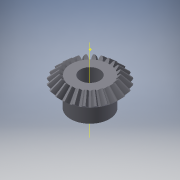
# Autodesk Inventor part: Bevel Gear2
Saved by Autodesk Inventor 2016 (Build 200138000, 138)
## iProperties
Created: 2015-06-13
Part Number: Bevel Gear2
Material: Steel, Mild
Document SubType Name: Modeling
Designer: steele
Categories: <?xml version="1.0" encoding="UTF-16"?> <MemberInstance><Categories><FamilyTemplate><FamilyTemplateParameter ValueType="xs:double" Id="1" ObjectReferenceKey="da_z" ObjectType="kUserParameterObject"/><FamilyTemplateParameter ValueType="xs:double" Id="2" ObjectReferenceKey="da_b" ObjectType="kUserParameterObject"/><FamilyTemplateParameter ValueType="xs:double" Id="3" ObjectReferenceKey="da_beta" ObjectType="kUserParameterObject"/><FamilyTemplateParameter ValueType="xs:double" Id="4" ObjectReferenceKey="da_dae" ObjectType="kUserParameterObject"/><FamilyTemplateParameter ValueType="xs:double" Id="5" ObjectReferenceKey="da_ve" ObjectType="kUserParameterObject"/><FamilyTemplateParameter ValueType="xs:double" Id="6" ObjectReferenceKey="da_omega" ObjectType="kUserParameterObject"/><FamilyTemplateParameter ValueType="xs:string" Id="7" ObjectReferenceKey="EAIAABAAAAAAHwAAAAAAAIAAAAAAAAAA" ObjectType="83914240" SubObjectId="SurfaceGeometry"/></FamilyTemplate><ParamToTemplateMap><ParamToTemplate CategoryParameter="//CategoryParameter[@InternalName='046C89C9-8512-4d59-83FE-43B91F4F132A']" TemplateParameter="1"/><ParamToTemplate CategoryParameter="//CategoryParameter[@InternalName='2552DF32-E462-4b46-AEBF-C6C7768E72AC']" TemplateParameter="2"/><ParamToTemplate CategoryParameter="//CategoryParameter[@InternalName='C9EE641D-15FC-4fae-A226-E94C4372FDD7']" TemplateParameter="3"/><ParamToTemplate><ParamToTemplate CategoryParameter="//CategoryParameter[@InternalName='00B6519A-459B-49c7-AD84-2E56D39A5744']" ConstantValue="-0.000000"/></ParamToTemplate><ParamToTemplate><ParamToTemplate CategoryParameter="//CategoryParameter[@InternalName='04B31F0E-C7A6-4894-AA32-9629BEFACF47']" ConstantValue="1.000000"/></ParamToTemplate><ParamToTemplate><ParamToTemplate CategoryParameter="//CategoryParameter[@InternalName='43CBEC2E-7847-49e7-A936-2F7889FCB2D9']" ConstantValue="0.200000"/></ParamToTemplate><ParamToTemplate><ParamToTemplate CategoryParameter="//CategoryParameter[@InternalName='B1EFC894-105D-4ebd-86BF-FA20ED196853']" ConstantValue="0.300000"/></ParamToTemplate><ParamToTemplate><ParamToTemplate CategoryParameter="//CategoryParameter[@InternalName='51175063-3D10-4879-93E8-6246FE8B403D']" ConstantValue="2061532430.657340"/></ParamToTemplate><ParamToTemplate><ParamToTemplate CategoryParameter="//CategoryParameter[@InternalName='A3A52E27-4454-46a9-B0BD-C932399B70AF']" ConstantValue="0.300000"/></ParamToTemplate><ParamToTemplate CategoryParameter="//CategoryParameter[@InternalName='2A200944-5A8C-41ca-B96E-8520D2E510F1']" TemplateParameter="4"/><ParamToTemplate><ParamToTemplate CategoryParameter="//CategoryParameter[@InternalName='1A637F62-92C8-44bc-B81F-10802510B579']" ConstantValue="2.855338"/></ParamToTemplate><ParamToTemplate CategoryParameter="//CategoryParameter[@InternalName='B52DD4BE-6863-48fb-BF58-89EF6F9EC65C']" TemplateParameter="5"/><ParamToTemplate><ParamToTemplate CategoryParameter="//CategoryParameter[@InternalName='3956BFF2-84D2-457d-93C2-9B0613DEBA67']" ConstantValue="1.268779"/></ParamToTemplate><ParamToTemplate CategoryParameter="//CategoryParameter[@InternalName='739CFA02-461B-4bf8-8049-181FCAD8B28F']" TemplateParameter="6"/><ParamToTemplate><ParamToTemplate CategoryParameter="//CategoryParameter[@InternalName='A27E999F-E2CE-4481-8A2A-EBF499C4C3C5']" ConstantValue="-0.000000"/></ParamToTemplate><ParamToTemplate><ParamToTemplate CategoryParameter="//CategoryParameter[@InternalName='9E1B4470-B2D3-4ff1-B813-535BB4CDF51A']" ConstantValue="3523220.976809"/></ParamToTemplate><ParamToTemplate><ParamToTemplate CategoryParameter="//CategoryParameter[@InternalName='F8452263-BFF6-458c-9FB1-07C4B99E95CD']" ConstantValue="11397033.805607"/></ParamToTemplate><ParamToTemplate><ParamToTemplate CategoryParameter="//CategoryParameter[@InternalName='3E3BB259-FD49-497f-8171-6EBC954A3479']" ConstantValue="2.000000"/></ParamToTemplate><ParamToTemplate CategoryParameter="//CategoryParameter[@InternalName='27C3BAF2-7550-4e4b-AE2C-0DB134B7D9B7']" TemplateParameter="7"/></ParamToTemplateMap><Category DisplayName="Gear" InternalName="DC85795E-93AB-48d5-8EEE-5A27447B64BD" Mnemonic="Gear"><CategoryParameter DisplayName="z" InternalName="046C89C9-8512-4d59-83FE-43B91F4F132A" Mnemonic="z"/><CategoryParameter DisplayName="b" InternalName="2552DF32-E462-4b46-AEBF-C6C7768E72AC" Mnemonic="b"/><CategoryParameter DisplayName="||b|" InternalName="C9EE641D-15FC-4fae-A226-E94C4372FDD7" Mnemonic="beta"/><CategoryParameter DisplayName="x" InternalName="00B6519A-459B-49c7-AD84-2E56D39A5744" Mnemonic="x"/><CategoryParameter DisplayName="a*" InternalName="04B31F0E-C7A6-4894-AA32-9629BEFACF47" Mnemonic="a"/><CategoryParameter DisplayName="c*" InternalName="43CBEC2E-7847-49e7-A936-2F7889FCB2D9" Mnemonic="c"/><CategoryParameter DisplayName="r|.f|*" InternalName="B1EFC894-105D-4ebd-86BF-FA20ED196853" Mnemonic="rf"/><CategoryParameter DisplayName="E" InternalName="51175063-3D10-4879-93E8-6246FE8B403D" Mnemonic="E"/><CategoryParameter DisplayName="||m|" InternalName="A3A52E27-4454-46a9-B0BD-C932399B70AF" Mnemonic="mi"/><Category DisplayName="BevelGear" InternalName="0C98F69A-0C2B-4791-B2FE-7691BB227E77" Mnemonic="BevelGear"><CategoryParameter DisplayName="d|.ae|" InternalName="2A200944-5A8C-41ca-B96E-8520D2E510F1" Mnemonic="dae"/><CategoryParameter DisplayName="d|.ai|" InternalName="1A637F62-92C8-44bc-B81F-10802510B579" Mnemonic="dai"/><CategoryParameter DisplayName="A|.e|" InternalName="B52DD4BE-6863-48fb-BF58-89EF6F9EC65C" Mnemonic="ve"/><CategoryParameter DisplayName="A|.i|" InternalName="3956BFF2-84D2-457d-93C2-9B0613DEBA67" Mnemonic="vi"/><CategoryParameter DisplayName="||S|" InternalName="739CFA02-461B-4bf8-8049-181FCAD8B28F" Mnemonic="omega"/><CategoryParameter DisplayName="x|.t|" InternalName="A27E999F-E2CE-4481-8A2A-EBF499C4C3C5" Mnemonic="xt"/><CategoryParameter DisplayName="||s||.Flim|" InternalName="9E1B4470-B2D3-4ff1-B813-535BB4CDF51A" Mnemonic="sFlim"/><CategoryParameter DisplayName="||s||.Hlim|" InternalName="F8452263-BFF6-458c-9FB1-07C4B99E95CD" Mnemonic="sHlim"/><CategoryParameter DisplayName="type" InternalName="3E3BB259-FD49-497f-8171-6EBC954A3479" Mnemonic="type"/><CategoryParameter DisplayName="PitchDiameter" InternalName="27C3BAF2-7550-4e4b-AE2C-0DB134B7D9B7" Mnemonic="IDS_PITCHDIAM"/></Category></Category></Categories></MemberInstance>
Mass: 60.9118 g
Surface Area: 34.3074 cm^2
Volume: 7.7496 cm^3
Density: 7.86 g/cm^3
Appearance: Steel
CustomPartVersion: 1
d48: 0.0000 in
d49: 0.0000 in
d50: 90.00 deg
d52: 0.0000 in
d53: 0.0000 in
d54: 0.00 deg
Author: steele
Autodesk Inventor part; units mm, degrees
ref_plane "Mesh Plane2" through (0, 0, 0) normal (0.9914449, 0.1305262, 0) x (0, 0, 1)
sketch "Teeth Body Sketch" plane through (0, 0, 0) normal (1, 0, 0) x (0, 1, 0)
  line L0 (0, 0) -> (17.702962, -20.397039) construction
  line L1 (17.702962, -20.397039) -> (20.172532, -17.927468)
  line L2 (20.172532, -17.927468) -> (0, 0) construction
  line L3 (19.05, -19.05) -> (0, 0) construction
  line L4 (12.528903, -14.43558) -> (14.27669, -12.687793)
  line L5 (17.702962, -20.397039) -> (12.528903, -14.43558)
  line L6 (20.172532, -17.927468) -> (14.27669, -12.687793)
  line L7 (0, -33.066314) -> (0, 5.511052)
  line L8 (0, -19.05) -> (20.172532, -19.05) construction
  dimension "d0" = 38.1
  dimension "d1" = 35.40592
  dimension "d2" = 40.34506
  dimension "d3" = 7.874
  dimension "d4" = 17.92747
  constraints: 16 end point, 4 point on line, 3 perpendicular, 2 collinear, 1 horizontal alignment, 1 vertical alignment
  measures "d0" diameter of L3.start L7
  measures "d1" diameter of L0.end L7
  measures "d2" diameter of L1.end L7
  measures "d3" distance between parallel lines of L1 L4
  measures "d4" vertical distance of L1.end L0.start
revolve "Teeth Body" add sketch "Teeth Body Sketch" angle 360 about axis through (0, 0, 0) along (0, 0, 1)
ref_plane "Tooth Plane" through (0, 19.05, -19.05) normal (0, -0.7071068, 0.7071068) x (1, 0, 0)
sketch "Start Sketch" plane through (0, 19.05, -19.05) normal (0, -0.7071068, 0.7071068) x (1, 0, 0)
  line L0 (0, -43.954783) -> (0, 12.281529)
  arc A0 (-0.600729, -2.3241) -> (-2.796445, 2.50275) centre (-10.245884, -3.798809) ccw
  arc A1 (2.796445, 2.50275) -> (0.600729, -2.3241) centre (10.245884, -3.798809) ccw
  line L1 (-0.600729, -2.3241) -> (0.600729, -2.3241)
  arc A2 (2.796445, 2.50275) -> (-2.796445, 2.50275) centre (0, -26.940768) ccw
  dimension "d7" = 9.75724
  dimension "d8" = 10.24588
  dimension "d9" = 23.14196
  dimension "d57" = 29.57602
  dimension "d58" = 24.61667
  constraints: 6 point on circle, 3 centre point, 3 symmetric about line, 2 end point, 1 coincident, 1 perpendicular, 1 other
  measures "d7" radius of A0
  measures "d8" horizontal distance of point (0, -26.941) A0.centre
  measures "d9" vertical distance of point (0, -26.941) A0.centre
  measures "d57" radius of A2
  measures "d58" distance from line of A2.centre L1
sketch "End Sketch" plane through (0, 13.358763, -13.358763) normal (0, -0.7071068, 0.7071068) x (1, 0, 0)
  line L0 (0, -28.080566) -> (0, 7.892027)
  arc A0 (-0.42186, -1.605152) -> (-1.963796, 1.78449) centre (-7.195145, -2.640763) ccw
  arc A1 (1.963796, 1.78449) -> (0.42186, -1.605152) centre (7.195145, -2.640763) ccw
  line L1 (-0.42186, -1.605152) -> (0.42186, -1.605152)
  arc A2 (1.963796, 1.78449) -> (-1.963796, 1.78449) centre (0, -18.892143) ccw
  dimension "d12" = 6.852
  dimension "d15" = 7.19514
  dimension "d16" = 16.25138
  dimension "d59" = 20.76968
  dimension "d60" = 17.28699
  constraints: 6 point on circle, 3 centre point, 3 symmetric about line, 2 end point, 1 coincident, 1 other
  measures "d12" radius of A0
  measures "d15" horizontal distance of A0.centre point (0, -18.892)
  measures "d16" vertical distance of A0.centre point (0, -18.892)
  measures "d59" radius of A2
  measures "d60" distance from line of A2.centre L1
loft "Loft" cut profiles "Start Sketch", "End Sketch"
pattern_circular "Circular Pattern" count 24 over 360 about axis through (0, 0, 0) along (0, 0, 1) of "Loft"
ref_plane "End Plane" through (0, 13.358763, -13.358763) normal (0, -0.7071068, 0.7071068) x (1, 0, 0)
sketch3d "3D Sketch Right"
ref_plane "End Plane Right" through (-1.865438, 13.227875, -13.358763) normal (0.0987415, -0.7001786, 0.7071068) x (0.9902021, 0.1396415, 0)
sketch "End Sketch Right" plane through (-1.865438, 13.227875, -13.358763) normal (0.0987415, -0.7001786, 0.7071068) x (0.9902021, 0.1396415, 0)
  arc A0 (-0.42186, -1.605152) -> (-1.963796, 1.78449) centre (-7.195145, -2.640763) ccw
  line L0 (0, -30.54214) -> (0, 10.353601)
  arc A1 (1.963796, 1.78449) -> (0.42186, -1.605152) centre (7.195145, -2.640763) ccw
  line L1 (-0.42186, -1.605152) -> (0.42186, -1.605152)
  arc A2 (1.963796, 1.78449) -> (-1.963796, 1.78449) centre (0, -18.892143) ccw
  dimension "d70" = 7.19514
  dimension "d71" = 16.25138
  dimension "d72" = 6.852
  dimension "d73" = 17.28699
  dimension "d74" = 20.76968
  constraints: 6 point on circle, 3 centre point, 3 symmetric about line, 2 end point, 1 coincident, 1 perpendicular, 1 other
  measures "d70" horizontal distance of A2.centre A0.centre
  measures "d71" vertical distance of point (0, -18.892) A0.centre
  measures "d72" radius of A0
  measures "d73" distance from line of point (0, -18.892) L1
  measures "d74" radius of A2
feature "Loft Right" [suppressed]
pattern_circular "Circular Pattern Right" [suppressed]
sketch3d "3D Sketch Left"
ref_plane "End Plane Left" through (1.907645, 13.227875, -13.372771) normal (-0.1009001, -0.6996557, 0.7073196) x (0.9897606, -0.1427373, 0)
sketch "End Sketch Left" plane through (1.907645, 13.227875, -13.372771) normal (-0.1009001, -0.6996557, 0.7073196) x (0.9897606, -0.1427373, 0)
  line L0 (0, -33.335466) -> (0, 12.869422)
  arc A0 (-0.42186, -1.599464) -> (-1.963796, 1.790178) centre (-7.195145, -2.635075) ccw
  arc A1 (1.963796, 1.790178) -> (0.42186, -1.599464) centre (7.195145, -2.635075) ccw
  line L1 (-0.42186, -1.599464) -> (0.42186, -1.599464)
  ellipse E0 centre (0, -8.968923) end of major axis (14.27669, -8.968923) minor radius 10.098183
  arc A2 (1.963796, 1.790178) -> (-1.963796, 1.790178) centre (0, -18.886455) ccw
  dimension "d56" = 10.09818
  dimension "d30" = 6.852
  dimension "d31" = 7.19514
  dimension "d32" = 16.25138
  dimension "d61" = 20.76968
  dimension "d62" = 17.28699
  constraints: 6 point on circle, 3 centre point, 3 symmetric about line, 2 end point, 1 coincident, 2 other
  measures "d30" radius of A0
  measures "d31" horizontal distance of point (0, -18.886) A0.centre
  measures "d32" vertical distance of A0.centre point (0, -18.886)
  measures "d61" radius of A2
  measures "d62" distance from line of point (0, -18.886) L1
feature "Loft Left" [suppressed]
pattern_circular "Circular Pattern Left" [suppressed]
sketch "Body Sketch" plane through (0, 0, 0) normal (1, 0, 0) x (0, 1, 0)
  line L0 (0, -29.503713) -> (0, -15.864554)
  line L1 (17.702962, -20.397039) -> (12.528903, -14.43558)
  line L2 (12.528903, -14.43558) -> (0, -14.43558)
  line L3 (17.702962, -20.397039) -> (0, -20.397039)
  constraints: 4 end point, 2 perpendicular, 2 point on line
sketch "Body Sketch outline for Fix Body" plane through (0, 0, 0) normal (1, 0, 0) x (0, 1, 0)
  line L0 (0, -20.397039) -> (17.702962, -20.397039)
  line L1 (0, -14.43558) -> (0, -20.397039)
  line L2 (12.528903, -14.43558) -> (0, -14.43558)
  line L3 (17.702962, -20.397039) -> (12.528903, -14.43558)
revolve "Fix Body" add sketch "Body Sketch outline for Fix Body" angle 360 about axis through (0, 0, 0) along (0, 0, 1)
sketch "Sketch6" plane through (0, 0, 0) normal (1, 0, 0) x (0, 1, 0)
  line L0 (19.05, -19.05) -> (0, 0) projected
  line L1 (0, -30.48) -> (0, 5.08) projected
surface revolve "Pitch Diameter" sketch "Sketch6" angle 360 about axis through (0, 0, 0) along (0, 0, 1) shown no curves L0
sketch "Sketch9" plane through (0, 0, -20.397039) normal (0, 0, -1) x (-1, 0, 0)
  circle A0 centre (0, 0) radius 12.7
  dimension "d95" = 25.4
  constraints: 1 centre point, 1 coincident
  measures "d95" diameter of A0
extrude "Extrusion2" add sketch "Sketch9" along normal blind 12.7
sketch "Sketch8" plane through (0, 0, -14.43558) normal (0, 0, 1) x (1, 0, 0)
  circle A0 centre (0, 0) radius 6.35
  dimension "d90" = 12.7
  constraints: 1 centre point, 1 coincident
  measures "d90" diameter of A0
extrude "Extrusion1" cut sketch "Sketch8" against normal through all
equation "\"d0\" = da_de"
equation "\"d1\" = da_dfe"
equation "\"d2\" = da_dae"
equation "\"d3\" = da_b"
equation "\"d4\" = da_ve"
equation "\"d7\" = fd_rr"
equation "\"d8\" = fd_x"
equation "\"d9\" = fd_y"
equation "\"d57\" = 0.5 * fd_dva + 0.3 * da_he"
equation "\"d58\" = 0.5 * fd_dva - 1.12 * da_he"
equation "\"da_teethtype\" = 0"
equation "\"da_b\" = 7.874"
equation "\"da_de\" = 38.1"
equation "\"da_dae\" = 40.34506"
equation "\"da_dfe\" = 35.40592"
equation "\"da_le\" = 26.94077"
equation "\"da_omega\" = 90deg"
equation "\"da_beta\" = 0"
equation "\"da_delta\" = 45deg"
equation "\"da_alpha\" = 20deg"
equation "\"da_he\" = 3.4925"
equation "\"da_ve\" = 17.92747"
equation "\"da_zv\" = 33.941125"
equation "\"fd_loft\" = da_b + 0.05 * da_he"
equation "\"fd_x\" = fd_x1 + fd_x2"
equation "\"fd_y\" = fd_y1 - fd_y2"
equation "\"fd_dd\" = fd_dva - 0.8 * da_he"
equation "\"da_dvw\" = 53.88154"
equation "\"d11\" = fd_loft"
equation "\"da_dm\" = 32.53224"
equation "\"da_x\" = 0"
equation "\"da_m\" = 1.5875"
equation "\"d50\" = da_omega"
equation "\"fd_rr\" = 9.757243"
equation "\"fd_dva\" = 57.056537"
equation "\"fd_x1\" = 1.246375"
equation "\"fd_x2\" = 8.999509"
equation "\"fd_y1\" = 26.911922"
equation "\"fd_y2\" = 3.769963"
body "Solid1"
body "Srf1"
